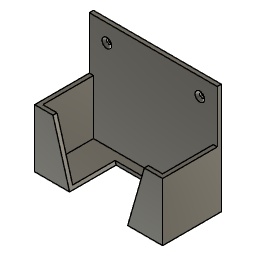
brickHolder v3 (Autodesk Fusion 360 design; units mm, degrees)
Autodesk Fusion 360 part; units mm, degrees
sketch "Sketch1" plane through (0, 0, 0) normal (0, 0, 1) x (1, 0, 0) in component "BrickHolder"
  line L0 (0, 0) -> (-110, 0)
  line L1 (-110, 0) -> (-110, 51)
  line L2 (-110, 51) -> (0, 51)
  line L3 (0, 51) -> (0, 0)
  dimension "d1" = 110
  dimension "d2" = 51
  constraint horizontal L0
  constraint vertical L1
  constraint horizontal L2
  constraint vertical L3
  constraint coincident L0.start L3.end
  measures "d1" distance of L0.start L0.end
  measures "d2" distance of L0.start L2.end
extrude "Extrude1" add sketch "Sketch1" along normal blind 95 in component "BrickHolder"
sketch "Sketch2" plane through (-110, 0, 0) normal (-1, 0, 0) x (0, -1, 0) in component "BrickHolder"
  line L0 (-51, 0) -> (0, 0)
  line L1 (0, 0) -> (0, 95)
  line L2 (0, 95) -> (-51, 95)
  line L3 (-51, 95) -> (-51, 0)
  line L4 (0, 95) -> (-47, 95)
  line L5 (-47, 95) -> (-47, 35)
  line L6 (-47, 35) -> (0, 35)
  line L7 (0, 35) -> (0, 95)
  dimension "d5" = 47
  dimension "d6" = 60
  constraint horizontal L4
  constraint vertical L5
  constraint horizontal L6
  constraint vertical L7
  constraint coincident L1.end L2.start
  measures "d5" distance of L1.end L4.end
  measures "d6" distance of L1.end L6.end
extrude "Extrude2" cut sketch "Sketch2" against normal blind 140 contours L1 L2 L4 L5 L6 L7 in component "BrickHolder"
sketch "Sketch3" plane through (0, 0, 35) normal (0, 0, 1) x (-1, 0, 0) in component "BrickHolder"
  line L0 (0, 0) -> (0, -47)
  line L1 (0, -47) -> (110, -47)
  line L2 (110, -47) -> (110, 0)
  line L3 (110, 0) -> (0, 0)
  line L4 (0, -47) -> (3.5, -47) construction
  line L5 (110, -47) -> (106.5, -47) construction
  line L6 (0, 0) -> (3.5, 0) construction
  line L7 (3.5, 0) -> (3.5, -3.5) construction
  line L8 (3.5, -3.5) -> (0, -3.5) construction
  line L9 (0, -3.5) -> (0, 0) construction
  line L10 (110, 0) -> (106.5, 0) construction
  line L11 (106.5, 0) -> (106.5, -3.5) construction
  line L12 (106.5, -3.5) -> (110, -3.5) construction
  line L13 (110, -3.5) -> (110, 0) construction
  line L14 (106.5, -47) -> (3.5, -47)
  line L15 (3.5, -47) -> (3.5, -3.5)
  line L16 (3.5, -3.5) -> (106.5, -3.5)
  line L17 (106.5, -3.5) -> (106.5, -47)
  dimension "d9" = 3.5
  dimension "d10" = 3.5
  dimension "d11" = 3.5
  dimension "d12" = 3.5
  dimension "d13" = 3.5
  dimension "d14" = 3.5
  constraint coincident L0.end L1.start
  constraint perpendicular L0 L4
  constraint horizontal L5
  constraint coincident L1.end L2.start
  constraint horizontal L6
  constraint vertical L7
  constraint horizontal L8
  constraint vertical L9
  constraint coincident L0.start L3.end
  constraint horizontal L10
  constraint vertical L11
  constraint horizontal L12
  constraint vertical L13
  constraint coincident L2.end L3.start
  constraint horizontal L14
  constraint vertical L15
  constraint horizontal L16
  constraint vertical L17
  measures "d9" distance of L0.end L4.end
  measures "d10" distance of L1.end L5.end
  measures "d11" distance of L0.start L6.end
  measures "d12" distance of L0.start L8.end
  measures "d13" distance of L2.end L10.end
  measures "d14" distance of L2.end L12.end
extrude "Extrude3" cut sketch "Sketch3" against normal blind 32 contours L1 L14 L15 L16 L17 in component "BrickHolder"
sketch "Sketch4" plane through (0, 0, 0) normal (0, -1, 0) x (1, 0, 0) in component "BrickHolder"
  line L0 (0, 35) -> (-110, 35)
  line L1 (-110, 35) -> (-110, 0)
  line L2 (-110, 0) -> (0, 0)
  line L3 (0, 0) -> (0, 35)
  line L4 (0, 0) -> (-30, 0) construction
  line L5 (-110, 35) -> (-90, 35) construction
  line L6 (0, 35) -> (-20, 35) construction
  line L7 (-110, 0) -> (-80, 0) construction
  line L8 (-90, 35) -> (-80, 0)
  line L9 (-30, 0) -> (-20, 35)
  line L10 (-20, 35) -> (-90, 35)
  line L11 (-80, 0) -> (-30, 0)
  dimension "d17" = 30
  dimension "d18" = 20
  dimension "d19" = 20
  dimension "d20" = 30
  constraint coincident L2.end L3.start
  constraint perpendicular L3 L4
  constraint coincident L0.end L1.start
  constraint perpendicular L1 L5
  constraint coincident L0.start L3.end
  constraint perpendicular L3 L6
  constraint coincident L1.end L2.start
  constraint perpendicular L1 L7
  measures "d17" distance of L2.end L4.end
  measures "d18" distance of L0.end L5.end
  measures "d19" distance of L0.start L6.end
  measures "d20" distance of L1.end L7.end
extrude "Extrude4" cut sketch "Sketch4" against normal blind 40 contours L0 L2 L8 L9 L10 L11 in component "BrickHolder"
sketch "Sketch5" plane through (0, 47, 0) normal (0, -1, 0) x (1, 0, 0) in component "BrickHolder"
  line L0 (0, 35) -> (0, 95)
  line L1 (0, 95) -> (-110, 95)
  line L2 (-110, 95) -> (-110, 35)
  line L3 (-110, 35) -> (-106.5, 35)
  line L4 (-106.5, 35) -> (-106.5, 3)
  line L5 (-106.5, 3) -> (-3.5, 3)
  line L6 (-3.5, 3) -> (-3.5, 35)
  line L7 (-3.5, 35) -> (0, 35)
  line L8 (-110, 95) -> (-95, 95) construction
  line L9 (-95, 95) -> (-95, 80) construction
  line L10 (-95, 80) -> (-110, 80) construction
  line L11 (-110, 80) -> (-110, 95) construction
  line L12 (0, 95) -> (-15, 95) construction
  line L13 (-15, 95) -> (-15, 80) construction
  line L14 (-15, 80) -> (0, 80) construction
  line L15 (0, 80) -> (0, 95) construction
  circle A0 centre (-95, 80) radius 2.125
  circle A1 centre (-15, 80) radius 2.125
  dimension "d23" = 15
  dimension "d24" = 15
  dimension "d25" = 15
  dimension "d26" = 15
  dimension "d27" = 4.25
  dimension "d28" = 4.25
  constraint horizontal L8
  constraint vertical L9
  constraint horizontal L10
  constraint vertical L11
  constraint coincident L1.end L2.start
  constraint horizontal L12
  constraint vertical L13
  constraint horizontal L14
  constraint vertical L15
  constraint coincident L0.end L1.start
  constraint coincident L9.end L10.start
  constraint coincident L13.end L14.start
  measures "d23" distance of L1.end L8.end
  measures "d24" distance of L1.end L10.end
  measures "d25" distance of L0.end L12.end
  measures "d26" distance of L0.end L14.end
  measures "d27" diameter of A0
  measures "d28" diameter of A1
extrude "Extrude5" cut sketch "Sketch5" against normal blind 45 contours A0 | A1 in component "BrickHolder"
chamfer "Chamfer1" distance 2 angle 45 2 edges at (-96.9812, 47, 80.7684) (-16.9812, 47, 80.7684) in component "BrickHolder"
move_face "OffsetFaces1" offset 15 1 faces at (-1.1667, 16.8333, 35) in component "BrickHolder"
move_face "OffsetFaces2" offset 15 1 faces at (-108.8333, 16.8333, 35) in component "BrickHolder"
move_face "OffsetFaces3" offset -0.5 1 faces at (-67.8917, 51, 26.1129) in component "BrickHolder"
component "BrickHolder" placed x (1, 0, 0) y (0, 1, 0) z (0, 0, 1) at (0, 0, 0)
